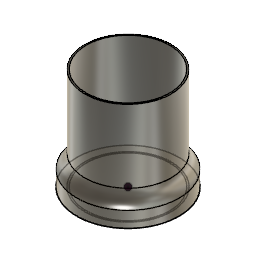
BladeMotorMount (Autodesk Fusion 360 design; units mm, degrees)
Autodesk Fusion 360 part; units mm, degrees
sketch "Sketch1" plane through (0, 0, 0) normal (0, 0, 1) x (1, 0, 0)
  circle A0 centre (0, 0) radius 32.5
  circle A1 centre (0, 0) radius 27.5
  circle A2 centre (0, 0) radius 26.5
  dimension "d1" = 65
  dimension "d2" = 55
  dimension "d3" = 53
  constraint coincident A0.centre A1.centre
  constraint concentric A0 A1
  measures "d1" diameter of A0
  measures "d2" diameter of A1
  measures "d3" diameter of A2
extrude "Extrude1" add sketch "Sketch1" along normal blind 10 contours A0
extrude "Extrude2" add sketch "Sketch1" along normal blind 65 contours A1
fillet "Fillet1" radius 10 1 edges at (-25.639, 9.9444, 10)
